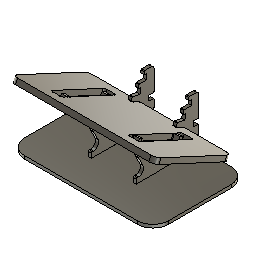
Stand2 (Autodesk Fusion 360 design; units mm, degrees)
Autodesk Fusion 360 part; units mm, degrees
sketch "スケッチ1" plane through (0, 0, 0) normal (0, 0, 1) x (1, 0, 0) in component "top1"
  line L0 (0, 0) -> (138, 0)
  line L1 (138, 0) -> (138, 80)
  line L2 (138, 80) -> (0, 80)
  line L3 (0, 80) -> (0, 0)
  line L4 (46.13, 80) -> (49, 80)
  line L5 (49, 80) -> (49, 74)
  line L6 (49, 74) -> (46.13, 74)
  line L7 (46.13, 74) -> (46.13, 80)
  line L8 (89, 80) -> (91.87, 80)
  line L9 (91.87, 80) -> (91.87, 74)
  line L10 (91.87, 74) -> (89, 74)
  line L11 (89, 74) -> (89, 80)
  line L12 (0, 80) -> (46.13, 74) construction
  line L13 (91.87, 74) -> (138, 80) construction
  line L14 (49, 74) -> (89, 74) construction
  line L15 (26.5, 68.87) -> (37.5, 68.87)
  line L16 (37.5, 68.87) -> (37.5, 11.13)
  line L17 (37.5, 11.13) -> (26.5, 11.13)
  line L18 (26.5, 11.13) -> (26.5, 68.87)
  line L19 (100.5, 68.87) -> (111.5, 68.87)
  line L20 (111.5, 68.87) -> (111.5, 11.13)
  line L21 (111.5, 11.13) -> (100.5, 11.13)
  line L22 (100.5, 11.13) -> (100.5, 68.87)
  line L23 (37.5, 62.87) -> (31.5, 62.87)
  line L24 (31.5, 62.87) -> (31.5, 60)
  line L25 (31.5, 60) -> (37.5, 60)
  line L26 (37.5, 60) -> (37.5, 62.87)
  line L27 (37.5, 20) -> (31.5, 20)
  line L28 (31.5, 20) -> (31.5, 17.13)
  line L29 (31.5, 17.13) -> (37.5, 17.13)
  line L30 (37.5, 17.13) -> (37.5, 20)
  line L31 (100.5, 62.87) -> (106.5, 62.87)
  line L32 (106.5, 62.87) -> (106.5, 60)
  line L33 (106.5, 60) -> (100.5, 60)
  line L34 (100.5, 60) -> (100.5, 62.87)
  line L35 (100.5, 20) -> (106.5, 20)
  line L36 (106.5, 20) -> (106.5, 17.13)
  line L37 (106.5, 17.13) -> (100.5, 17.13)
  line L38 (100.5, 17.13) -> (100.5, 20)
  line L39 (0, 80) -> (26.5, 68.87) construction
  line L40 (111.5, 68.87) -> (138, 80) construction
  line L41 (26.5, 11.13) -> (0, 0) construction
  line L42 (111.5, 11.13) -> (138, 0) construction
  line L43 (37.5, 62.57) -> (37.2, 62.57)
  line L44 (37.2, 62.57) -> (37.2, 60.3)
  line L45 (37.2, 60.3) -> (37.5, 60.3)
  line L46 (37.5, 60.3) -> (37.5, 62.57)
  line L47 (37.5, 19.7) -> (37.2, 19.7)
  line L48 (37.2, 19.7) -> (37.2, 17.43)
  line L49 (37.2, 17.43) -> (37.5, 17.43)
  line L50 (37.5, 17.43) -> (37.5, 19.7)
  line L51 (100.5, 62.57) -> (100.8, 62.57)
  line L52 (100.8, 62.57) -> (100.8, 60.3)
  line L53 (100.8, 60.3) -> (100.5, 60.3)
  line L54 (100.5, 60.3) -> (100.5, 62.57)
  line L55 (100.5, 19.7) -> (100.8, 19.7)
  line L56 (100.8, 19.7) -> (100.8, 17.43)
  line L57 (100.8, 17.43) -> (100.5, 17.43)
  line L58 (100.5, 17.43) -> (100.5, 19.7)
  dimension "d1" = 138
  dimension "d2" = 80
  dimension "d52" = 2.87
  dimension "d53" = 6
  dimension "d54" = 40
  dimension "d163" = 40
  dimension "d164" = 40
  dimension "d165" = 2.87
  dimension "d166" = 6
  dimension "d167" = 5
  dimension "d169" = 6
  dimension "d170" = 6
  dimension "d175" = 0.3
  dimension "d176" = 0.3
  dimension "d177" = 0.3
  dimension "d178" = 0.3
  dimension "d191" = 85
  constraint horizontal L0
  constraint vertical L1
  constraint horizontal L2
  constraint vertical L3
  constraint coincident L0.start L3.end
  constraint horizontal L4
  constraint vertical L5
  constraint horizontal L6
  constraint vertical L7
  constraint coincident L2 L4.start
  constraint horizontal L8
  constraint vertical L9
  constraint horizontal L10
  constraint vertical L11
  constraint coincident L2 L8.start
  constraint equal L5 L11
  constraint equal L6 L10
  constraint equal L12 L13
  constraint horizontal L15
  constraint vertical L16
  constraint horizontal L17
  constraint vertical L18
  constraint horizontal L19
  constraint vertical L20
  constraint horizontal L21
  constraint vertical L22
  constraint horizontal L23
  constraint vertical L24
  constraint horizontal L25
  constraint vertical L26
  constraint coincident L16 L23.start
  constraint horizontal L27
  constraint vertical L28
  constraint horizontal L29
  constraint vertical L30
  constraint coincident L16 L27.start
  constraint horizontal L31
  constraint vertical L32
  constraint horizontal L33
  constraint vertical L34
  constraint coincident L22 L31.start
  constraint horizontal L35
  constraint vertical L36
  constraint horizontal L37
  constraint vertical L38
  constraint coincident L22 L35.start
  constraint equal L25 L29
  constraint equal L24 L28
  constraint equal L24 L32
  constraint equal L32 L36
  constraint equal L33 L35
  constraint collinear L23 L31
  constraint collinear L15 L19
  constraint collinear L17 L21
  constraint equal L15 L19
  constraint equal L39 L40
  constraint equal L39 L41
  constraint equal L23 L31
  constraint horizontal L43
  constraint vertical L44
  constraint horizontal L45
  constraint vertical L46
  constraint coincident L26 L43.start
  constraint horizontal L47
  constraint vertical L48
  constraint horizontal L49
  constraint vertical L50
  constraint coincident L30 L47.start
  constraint horizontal L51
  constraint vertical L52
  constraint horizontal L53
  constraint vertical L54
  constraint coincident L34 L51.start
  constraint horizontal L55
  constraint vertical L56
  constraint horizontal L57
  constraint vertical L58
  constraint coincident L22 L55.start
  constraint collinear L44 L48
  constraint collinear L43 L51
  constraint collinear L45 L53
  constraint collinear L52 L56
  constraint collinear L47 L55
  constraint collinear L49 L57
  constraint equal L44 L48
  constraint equal L43 L51
  measures "d1" distance of L0.start L0.end
  measures "d2" distance of L0.start L2.end
  measures "d52" distance of L5.end L6.end
  measures "d53" distance of L4.start L6.end
  measures "d54" distance of L5.end L10.end
  measures "d163" distance of L25 L27
  measures "d164" distance of L33 L35
  measures "d165" distance of L23.end L24.end
  measures "d166" distance of L23.start L23.end
  measures "d167" distance of L18 L24
  measures "d169" distance of L15 L23
  measures "d170" distance of L17 L29
  measures "d175" distance of L23 L43
  measures "d176" distance of L25 L45
  measures "d177" distance of L26 L44
  measures "d178" distance of L29 L49
  measures "d191" distance of L18 L20
extrude "押し出し1" add sketch "スケッチ1" along normal blind 5 contours L0 L1 L2 L3 L5 L6 L7 L9 L10 L11 | L16 L23 L24 L25 L26 L43 L44 L45 | L16 L27 L28 L29 L30 L47 L48 L49 | L22 L31 L32 L33 L34 L51 L52 L53 | L22 L35 L36 L37 L38 L55 L56 L57 makes body 1 in component "top1"
sketch "スケッチ1 (2)" plane through (0, 0, 0) normal (0, 0, 1) x (1, 0, 0) in component "base1"
  line L0 (-147.4863, 0.0694) -> (-9.4863, 0.0694)
  line L1 (-9.4863, 0.0694) -> (-9.4863, 90.0694)
  line L2 (-9.4863, 90.0694) -> (-147.4863, 90.0694)
  line L3 (-147.4863, 90.0694) -> (-147.4863, 0.0694)
  line L4 (-101.3563, 67.5694) -> (-98.4863, 67.5694)
  line L5 (-98.4863, 67.5694) -> (-98.4863, 52.5694)
  line L6 (-98.4863, 52.5694) -> (-101.3563, 52.5694)
  line L7 (-101.3563, 52.5694) -> (-101.3563, 67.5694)
  line L8 (-58.4863, 67.5694) -> (-55.6163, 67.5694)
  line L9 (-55.6163, 67.5694) -> (-55.6163, 52.5694)
  line L10 (-55.6163, 52.5694) -> (-58.4863, 52.5694)
  line L11 (-58.4863, 52.5694) -> (-58.4863, 67.5694)
  line L12 (-101.3563, 60.0694) -> (-148.1899, 60.0694) construction
  line L13 (-55.6163, 60.0694) -> (-8.7828, 60.1949) construction
  line L14 (-98.4863, 60.0694) -> (-58.4863, 60.0694) construction
  line L15 (-147.4863, 90.0694) -> (-101.3563, 67.5694) construction
  line L16 (-55.6163, 67.5694) -> (-9.4863, 90.0694) construction
  dimension "d5" = 138
  dimension "d6" = 90
  dimension "d45" = 15
  dimension "d46" = 2.87
  dimension "d47" = 40
  dimension "d99" = 30
  constraint horizontal L0
  constraint vertical L1
  constraint horizontal L2
  constraint vertical L3
  constraint horizontal L4
  constraint vertical L5
  constraint horizontal L6
  constraint vertical L7
  constraint horizontal L8
  constraint vertical L9
  constraint horizontal L10
  constraint vertical L11
  constraint equal L5 L11
  constraint equal L4 L8
  constraint midpoint L7 L12.start
  constraint midpoint L9 L13.start
  constraint midpoint L5 L14.start
  constraint midpoint L11 L14.end
  constraint horizontal L12
  constraint horizontal L14
  constraint equal L12 L13
  constraint equal L15 L16
  measures "d5" distance of L0.start L0.end
  measures "d6" distance of L0.start L2.end
  measures "d45" distance of L4.start L6.end
  measures "d46" distance of L4.start L4.end
  measures "d47" distance of L14.start L14.end
  measures "d99" distance of L2 L12
extrude "押し出し1'" add sketch "スケッチ1 (2)" along normal blind 3 separate body makes body 2 in component "base1"
sketch "スケッチ1 (3)" plane through (0, 0, 0) normal (1, 0, 0) x (0, 1, 0) in component "leg1"
  line L0 (92.2311, 6.6468) -> (152.2311, 6.6468)
  line L1 (152.2311, 6.6468) -> (152.2311, 54.0023)
  line L2 (137.969, 45.4523) -> (92.2311, 45.4523) construction
  line L3 (92.2311, 45.4523) -> (92.2311, 6.6468)
  line L4 (114.7311, 6.6468) -> (129.7311, 6.6468)
  line L5 (129.7311, 6.6468) -> (129.7311, 3.7768)
  line L6 (129.7311, 3.7768) -> (114.7311, 3.7768)
  line L7 (114.7311, 3.7768) -> (114.7311, 6.6468)
  line L8 (122.2311, 3.7768) -> (122.2311, 6.6468) construction
  line L9 (88.1807, 52.0182) -> (96.3789, 44.8323) construction
  line L10 (82.9228, 51.1896) -> (123.6824, 32.27) construction
  line L11 (96.3789, 44.8323) -> (119.9267, 24.1924)
  line L12 (119.9267, 24.1924) -> (123.2225, 27.9525)
  line L13 (123.2225, 27.9525) -> (121.3424, 29.6003)
  line L14 (123.6824, 32.27) -> (130.2694, 29.2125)
  line L15 (130.2694, 29.2125) -> (132.3746, 33.7477)
  line L16 (132.3746, 33.7477) -> (130.1069, 34.8003)
  line L17 (92.2311, 46.0107) -> (131.6016, 38.0203) construction
  line L18 (131.6016, 38.0203) -> (138.7185, 36.5759)
  line L19 (138.7185, 36.5759) -> (139.713, 41.476)
  line L20 (139.713, 41.476) -> (137.263, 41.9732)
  circle A0 centre (94.7311, 42.9523) radius 2.5
  line L21 (121.3424, 29.6003) -> (123.6824, 32.27)
  line L22 (130.1069, 34.8003) -> (131.6016, 38.0203)
  line L23 (137.263, 41.9732) -> (137.969, 45.4523)
  circle A1 centre (147.4925, 16.3968) radius 3.25
  line L24 (152.2311, 18.1468) -> (150.2311, 18.1468)
  line L25 (150.2311, 18.1468) -> (150.2311, 14.6468)
  line L26 (150.2311, 14.6468) -> (152.2311, 14.6468)
  line L27 (152.2311, 14.6468) -> (152.2311, 18.1468)
  line L28 (152.2311, 54.0023) -> (142.7311, 54.0023)
  line L29 (142.7311, 54.0023) -> (142.7311, 50.4523)
  line L30 (142.7311, 50.4523) -> (145.2311, 50.4523)
  line L31 (145.2311, 50.4523) -> (145.2311, 45.4523)
  line L32 (137.969, 45.4523) -> (145.2311, 45.4523)
  line L33 (123.6824, 32.27) -> (142.7311, 54.0023) construction
  line L34 (131.6016, 38.0203) -> (142.5726, 61.6557) construction
  line L35 (137.969, 45.4523) -> (141.6214, 63.4486) construction
  line L36 (92.2311, 31.6468) -> (102.2311, 11.6468)
  line L37 (102.2311, 11.6468) -> (92.2311, 11.6468)
  line L38 (152.2311, 31.5968) -> (147.2311, 31.5968)
  line L39 (147.2311, 31.5968) -> (147.2311, 26.6468)
  line L40 (147.2311, 26.6468) -> (152.2311, 26.6468)
  line L41 (152.2311, 26.6468) -> (152.2311, 31.5968)
  dimension "d16" = 15
  dimension "d17" = 2.87
  dimension "d40" = 60
  dimension "d68" = 5
  dimension "d95" = 3.55
  dimension "d115" = 6.5
  dimension "d117" = 2
  dimension "d118" = 8
  dimension "d119" = 3.5
  dimension "d126" = 7
  dimension "d132" = 2.5
  dimension "d162" = 5
  dimension "d179" = 10
  dimension "d180" = 20
  dimension "d181" = 5
  dimension "d188" = 4.95
  dimension "d189" = 5
  dimension "d190" = 20
  constraint horizontal L0
  constraint vertical L1
  constraint horizontal L2
  constraint vertical L3
  constraint coincident L3 L17.start
  constraint horizontal L4
  constraint vertical L5
  constraint horizontal L6
  constraint vertical L7
  constraint coincident L0 L4.start
  constraint midpoint L6 L8.start
  constraint midpoint L0 L8.end
  constraint vertical L8
  constraint perpendicular L9 L12
  constraint collinear L9 L11
  constraint perpendicular L14 L15
  constraint perpendicular L15 L16
  constraint collinear L10 L14
  constraint equal L12 L15
  constraint equal L13 L16
  constraint coincident L2 L23.end
  constraint perpendicular L18 L19
  constraint perpendicular L19 L20
  constraint collinear L17 L18
  constraint perpendicular L12 L13
  constraint tangent L3 A0
  constraint tangent L2 A0
  constraint tangent L9 A0
  constraint tangent L10 A0
  constraint tangent L17 A0
  constraint coincident L10 L14.start
  constraint perpendicular L20 L23
  constraint perpendicular L16 L22
  constraint perpendicular L13 L21
  constraint equal L21 L22
  constraint coincident L17.end L18.start
  constraint equal L15 L19
  constraint equal L22 L23
  constraint equal L16 L20
  constraint horizontal L24
  constraint vertical L25
  constraint horizontal L26
  constraint vertical L27
  constraint coincident A1 L25.end
  constraint coincident L1 L24.start
  constraint coincident A1 L24.end
  constraint perpendicular L1 L28
  constraint perpendicular L28 L29
  constraint perpendicular L29 L30
  constraint coincident L2 L31.end
  constraint perpendicular L2 L31
  constraint equal L23 L29
  constraint equal L19 L31
  constraint equal L20 L30
  constraint coincident L10.end L14.start
  constraint equal L18 L32
  constraint equal L14 L18
  constraint collinear L21 L33
  constraint coincident L9.end A0
  constraint coincident L28.end L29.start
  constraint parallel L22 L34
  constraint parallel L23 L35
  constraint coincident L3 L36.start
  constraint coincident L3 L37.end
  constraint horizontal L37
  constraint horizontal L38
  constraint vertical L39
  constraint horizontal L40
  constraint vertical L41
  constraint coincident L1 L38.start
  measures "d16" distance of L4.start L4.end
  measures "d17" distance of L4.start L6.end
  measures "d40" distance of L0.start L0.end
  measures "d68" diameter of A0
  measures "d95" distance of L20.end L2.start
  measures "d115" diameter of A1
  measures "d117" distance of L24.start L24.end
  measures "d118" distance of L0 L26
  measures "d119" distance of L24.end L25.end
  measures "d126" distance of L1 L31
  measures "d132" distance of L29.end L30.end
  measures "d162" distance of L11.end L12.end
  measures "d179" distance of L36.end L37.end
  measures "d180" distance of L36.start L37
  measures "d181" distance of L0 L37
  measures "d188" distance of L38.end L39.end
  measures "d189" distance of L39.end L40.end
  measures "d190" distance of L0 L40
extrude "押し出し1''" add sketch "スケッチ1 (3)" along normal blind 3 separate body contours L0 L1 L3 L4 L11 L12 L13 L14 L15 L16 L18 L19 L20 A0 L21 L22 L23 A1 L24 L26 L28 L29 L30 L31 L32 L36 L37 L38 L39 L40 | L0 L4 L5 L6 L7 | A0 makes body 3 in component "leg1"
fillet "フィレット1" radius 15 4 edges at (-147.4863, 0.0694, 1.5) (-9.4863, 0.0694, 1.5) (-147.4863, 90.0694, 1.5) (-9.4863, 90.0694, 1.5) on bodies 2 in component "base1"
fillet "フィレット1'" radius 5 4 edges at (0, 0, 2.5) (0, 80, 2.5) (138, 0, 2.5) (138, 80, 2.5) on bodies 1 in component "top1"
fillet "フィレット1'" radius 0.5 4 edges at (46.13, 80, 2.5) (49, 80, 2.5) (89, 80, 2.5) (91.87, 80, 2.5) on bodies 1 in component "top1"
fillet "フィレット1'" radius 2 8 edges at (111.5, 11.13, 2.5) (111.5, 68.87, 2.5) (100.5, 11.13, 2.5) (100.5, 68.87, 2.5) (37.5, 11.13, 2.5) (26.5, 11.13, 2.5) (26.5, 68.87, 2.5) (37.5, 68.87, 2.5) on bodies 1 in component "top1"
fillet "フィレット1'" radius 0.5 8 edges at (37.5, 17.13, 2.5) (37.5, 20, 2.5) (37.5, 60, 2.5) (37.5, 62.87, 2.5) (100.5, 17.13, 2.5) (100.5, 20, 2.5) (100.5, 60, 2.5) (100.5, 62.87, 2.5) on bodies 1 in component "top1"
fillet "フィレット2" radius 0.5 2 edges at (1.5, 152.2311, 18.1468) (1.5, 152.2311, 14.6468) on bodies 3 in component "leg1"
fillet "フィレット2" radius 0.5 2 edges at (1.5, 150.2311, 18.1468) (1.5, 150.2311, 14.6468) on bodies 3 in component "leg1"
fillet "フィレット2" radius 0.5 2 edges at (1.5, 129.7311, 3.7768) (1.5, 114.7311, 3.7768) on bodies 3 in component "leg1"
fillet "フィレット2" radius 0.5 8 edges at (1.5, 142.7311, 54.0023) (1.5, 142.7311, 50.4523) (1.5, 137.969, 45.4523) (1.5, 137.263, 41.9732) (1.5, 131.6016, 38.0203) (1.5, 130.1069, 34.8003) (1.5, 123.6824, 32.27) (1.5, 121.3424, 29.6003) on bodies 3 in component "leg1"
fillet "フィレット2" radius 2 1 edges at (1.5, 152.2311, 54.0023) on bodies 3 in component "leg1"
fillet "フィレット2" radius 5 1 edges at (1.5, 102.2311, 11.6468) on bodies 3 in component "leg1"
fillet "フィレット2" radius 1 1 edges at (1.5, 92.2311, 11.6468) on bodies 3 in component "leg1"
fillet "フィレット2" radius 20 1 edges at (1.5, 92.2311, 31.6468) on bodies 3 in component "leg1"
fillet "フィレット2" radius 0.5 2 edges at (1.5, 152.2311, 31.5968) (1.5, 152.2311, 26.6468) on bodies 3 in component "leg1"
sketch "スケッチ1 (4)" plane through (0, 0, 0) normal (0, 0, 1) x (1, 0, 0) in component "bridge1"
  line L0 (6.4862, 47.0082) -> (66.2262, 47.0082)
  line L1 (66.2262, 47.0082) -> (66.2262, 36.0082)
  line L2 (66.2262, 36.0082) -> (6.4862, 36.0082)
  line L3 (6.4862, 36.0082) -> (6.4862, 47.0082)
  line L4 (13.4862, 47.0082) -> (16.3562, 47.0082)
  line L5 (16.3562, 47.0082) -> (16.3562, 41.0082)
  line L6 (16.3562, 41.0082) -> (13.4862, 41.0082)
  line L7 (13.4862, 41.0082) -> (13.4862, 47.0082)
  line L8 (56.3562, 47.0082) -> (59.2262, 47.0082)
  line L9 (59.2262, 47.0082) -> (59.2262, 41.0082)
  line L10 (59.2262, 41.0082) -> (56.3562, 41.0082)
  line L11 (56.3562, 41.0082) -> (56.3562, 47.0082)
  dimension "d145" = 40
  dimension "d146" = 6
  dimension "d147" = 2.87
  dimension "d148" = 5
  dimension "d149" = 7
  dimension "d159" = 7
  dimension "d160" = 59.74
  constraint horizontal L0
  constraint vertical L1
  constraint horizontal L2
  constraint vertical L3
  constraint horizontal L4
  constraint vertical L5
  constraint horizontal L6
  constraint vertical L7
  constraint coincident L0 L4.start
  constraint horizontal L8
  constraint vertical L9
  constraint horizontal L10
  constraint vertical L11
  constraint coincident L0 L8.start
  constraint equal L5 L9
  constraint equal L6 L10
  measures "d145" horizontal distance of L5.end L10.end
  measures "d146" distance of L4.end L5.end
  measures "d147" distance of L4.start L4.end
  measures "d148" distance of L2 L10
  measures "d149" distance of L1 L9
  measures "d159" distance of L3 L7
  measures "d160" distance of L1.end L2.end
extrude "押し出し1'''" add sketch "スケッチ1 (4)" along normal blind 3 separate body contours L0 L1 L2 L3 L5 L6 L7 L9 L10 L11 makes body 4 in component "bridge1"
fillet "フィレット1''" radius 2 4 edges at (6.4862, 47.0082, 1.5) (6.4862, 36.0082, 1.5) (66.2262, 36.0082, 1.5) (66.2262, 47.0082, 1.5) on bodies 4 in component "bridge1"
fillet "フィレット1''" radius 0.5 4 edges at (13.4862, 47.0082, 1.5) (16.3562, 47.0082, 1.5) (56.3562, 47.0082, 1.5) (59.2262, 47.0082, 1.5) on bodies 4 in component "bridge1"
component "top1" placed x (1, 0, 0) y (0, 0.907047, -0.421029) z (0, 0.421029, 0.907047) at (-147.4213, 0.9862, 56.5918)
component "base1" placed x (1, 0, 0) y (0, 1, 0) z (0, 0, 1) at (0, 0, 0)
component "leg1" placed x (1, 0, 0) y (0, 1, 0) z (0, 0, 1) at (-58.4863, -62.1617, -3.7768)
component "leg1" placed x (1, 0, 0) y (0, 1, 0) z (0, 0, 1) at (-101.4863, -62.1617, -3.7768)
component "bridge1" placed x (1, 0, 0) y (0, 1, 0) z (0, 0, 1) at (0, 0, 0)
equation "d5 = d1"
equation "d16 = d45"
equation "d17 = d46"
equation "d40 = d99 * 2"
equation "d46 = d52"
equation "d47 = d54"
equation "d115 = d119 + 3 mm"
equation "d145 = d54"
equation "d146 = d53"
equation "d147 = d52"
equation "d159 = d149"
equation "d163 = d54"
equation "d164 = d163"
equation "d165 = d52"
equation "d166 = d53"
equation "d170 = d169"
equation "d176 = d175"
equation "d178 = d175"
equation "d189 = d167"
